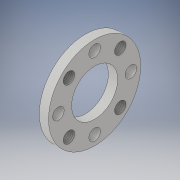
# Autodesk Inventor part: Robot Flange
Saved by Autodesk Inventor 2019 (Build 230136000, 136)
## iProperties
Created: 2019-06-10
Part Number: Robot Flange
Material: Generic
Document SubType Name: Modeling
Designer: Matthew XPS
Density: 1 g/cm^3
Appearance: Default
Author: Matthew XPS
Autodesk Inventor part; units mm, degrees
ref_plane "YZ Plane" through (0, 0, 0) normal (1, 0, 0) x (0, 1, 0)
ref_plane "XZ Plane" through (0, 0, 0) normal (0, 1, 0) x (-1, 0, 0)
ref_plane "XY Plane" through (0, 0, 0) normal (0, 0, 1) x (1, 0, 0)
sketch "Sketch1" plane through (0, 0, 0) normal (1, 0, 0) x (0, 1, 0)
  circle A0 centre (0, 0) radius 10
  circle A1 centre (0, 0) radius 20
  dimension "d0" = 20
  dimension "d3" = 40
  constraints: 2 centre point, 2 coincident
  measures "d0" diameter of A0
  measures "d3" diameter of A1
extrude "Extrusion1" add sketch "Sketch1" along normal blind 4
sketch "Sketch3" plane through (4, 0, 0) normal (1, 0, 0) x (0, 0, -1)
  line L0 (0, 0) -> (15.75, 0)
  circle A0 centre (15.75, 0) radius 2.5
  dimension "d4" = 15.75
  dimension "d5" = 5
  constraints: 2 end point, 1 centre point, 1 coincident, 1 horizontal
  measures "d4" distance of L0.start L0.end
  measures "d5" diameter of A0
extrude "Extrusion2" cut sketch "Sketch3" against normal blind 4
pattern_circular "Circular Pattern1" count 4 over 360 about axis through (-10, 0, 0) along (1, 0, 0) of "Extrusion2"
sketch "Sketch4" plane through (4, 0, 0) normal (1, 0, 0) x (0, 0, -1)
  line L0 (0, 0) -> (11.1369, 11.1369)
  line L1 (0, 0) -> (15.75, 0) construction
  circle A0 centre (11.1369, 11.1369) radius 2.5
  dimension "d11" = 15.75
  dimension "d12" = 45
  dimension "d13" = 5
  constraints: 4 end point, 1 centre point, 1 coincident, 1 equal length, 1 horizontal
  measures "d11" distance of L0.start L0.end
  measures "d12" angle of L1 L0
  measures "d13" diameter of A0
extrude "Extrusion3" cut sketch "Sketch4" against normal blind 4
thread "Thread1" size "M5x0.8" class "6H" standard "ANSI Metric M Profile" full length
pattern_circular "Circular Pattern2" count 4 over 360 about axis through (-10, 0, 0) along (1, 0, 0) of "Extrusion3"
body "Solid1"
